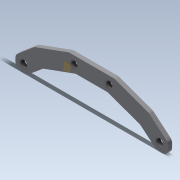
# Autodesk Inventor part: HeadTopConnector
Saved by Autodesk Inventor 2020 (Build 240168000, 168)
## iProperties
Created: 2021-07-09
Part Number: HeadTopConnector
Material: Generic
Document SubType Name: Sheet Metal
Designer: Val
Density: 1 g/cm^3
Sheet Metal Rule: Default
Appearance: Default
Author: Val
Autodesk Inventor part; units mm, degrees
ref_plane "YZ Plane" through (0, 0, 0) normal (1, 0, 0) x (0, 1, 0)
ref_plane "XZ Plane" through (0, 0, 0) normal (0, 1, 0) x (-1, 0, 0)
ref_plane "XY Plane" through (0, 0, 0) normal (0, 0, 1) x (1, 0, 0)
sketch "Base" plane through (0, 0, 0) normal (0, 0, 1) x (1, 0, 0)
  circle A0 centre (-46.4246, 117.9827) radius 2.5
  line L0 (-52.4246, 120.7805) -> (-52.4246, 111.9827)
  line L1 (-52.4246, 111.9827) -> (-44.2408, 111.9827)
  line L2 (-52.4246, 120.7805) -> (-44.8558, 127.1315)
  line L3 (-44.8558, 127.1315) -> (-16.5235, 137.4436)
  line L4 (-44.2408, 111.9827) -> (-38.7633, 116.5789)
  line L5 (-38.7633, 116.5789) -> (-11.6601, 126.4436)
  line L6 (-11.6601, 126.4436) -> (0.0157, 126.4436)
  line L7 (-16.5235, 137.4436) -> (0, 137.4436)
  line L8 (0.0001, 252.4162) -> (0.0001, -227.6975)
  line L9 (52.4249, 120.7805) -> (52.4249, 111.9827)
  line L10 (52.4249, 111.9827) -> (44.2411, 111.9827)
  line L11 (52.4249, 120.7805) -> (44.8561, 127.1315)
  line L12 (44.2411, 111.9827) -> (38.7635, 116.5789)
  line L13 (38.7635, 116.5789) -> (11.6604, 126.4436)
  line L14 (11.6604, 126.4436) -> (0.0157, 126.4436)
  line L15 (16.5238, 137.4436) -> (0, 137.4436)
  line L16 (16.5238, 137.4436) -> (44.8561, 127.1315)
  ellipse E0 centre (-12.7181, 132.4436) end of major axis (-10.7181, 132.4436) minor radius 1.9897
  ellipse E1 centre (12.7183, 132.4436) end of major axis (14.7183, 132.4436) minor radius 1.9897
  circle A1 centre (-46.4246, 117.9827) radius 3.175
  circle A2 centre (46.4246, 117.9827) radius 3.175
  point P0 (0, 0)
  dimension "d1" = 5
  dimension "d2" = 6
  dimension "d3" = 6
  dimension "d5" = 12
  dimension "d6" = 160
  dimension "d7" = 160
  dimension "d8" = 6
  dimension "d9" = 6
  dimension "d10" = 6
  dimension "d11" = 6
  dimension "d20" = 5
  measures "d1" distance from line of L7 E0.centre
  measures "d2" distance from line of L3 E0.centre
  measures "d3" distance from line of L6 E0.centre
  measures "d5" distance between parallel lines of L5 L3
  measures "d6" angle of L5 L4
  measures "d7" angle of L6 L5
  measures "d8" distance from line of L0 A0.centre
  measures "d9" distance from line of L2 A0.centre
  measures "d10" distance from line of L4 A0.centre
  measures "d11" distance from line of L1 A0.centre
  measures "d20" diameter of A0
extrude "Plate1" add sketch "Base" along normal blind 3.048 contours L2 L3 L7 L8 L6 L5 L4 L1 L0 | L15 L16 L11 L9 L10 L12 L13 L14 L6 L8
fillet "FilletsFeature" radius 4 14 edges at (-44.8558, 127.1315, 1.524) (-16.5235, 137.4436, 1.524) (-52.4246, 120.7805, 1.524) (-52.4246, 111.9827, 1.524) (16.5238, 137.4436, 1.524) (44.8561, 127.1315, 1.524) (52.4249, 120.7805, 1.524) (52.4249, 111.9827, 1.524) (44.2411, 111.9827, 1.524) (38.7635, 116.5789, 1.524) (11.6604, 126.4436, 1.524) (-11.6601, 126.4436, 1.524) (-38.7633, 116.5789, 1.524) (-44.2408, 111.9827, 1.524)
ref_plane "BentCutPlane" through (-12.7181, 132.4436, 8.3161) normal (0, 0.1014104, 0.9948447) x (0, -0.9948447, 0.1014104)
sketch "BentCutProfile" plane through (-12.7181, 132.4436, 8.3161) normal (0, 0.1014104, 0.9948447) x (0, -0.9948447, 0.1014104)
  circle A0 centre (0, 0) radius 2 projected
  circle A1 centre (0, 25.4364) radius 2 projected
  point P0 (130.9175, 12.7181)
hole "BentCutProfileHoleFeature" at (-12.7181, 132.4436, 8.3161) at (12.7183, 132.4436, 8.3161) direction (0, -0.1014104, -0.9948447) diameter 4.5 end through all
equation "\"d18\" = Thickness"
equation "\"d0\" = Thickness"
equation "\"BendRadius\" = Thickness"
equation "\"BendReliefWidth\" = Thickness"
equation "\"BendReliefDepth\" = 0.5 * Thickness"
equation "\"CornerReliefSize\" = 4 * Thickness"
equation "\"MinimumRemnant\" = 2 * Thickness"
equation "\"TransitionRadius\" = BendRadius"
equation "\"JacobiRadiusSize\" = BendRadius"
equation "\"GapSize\" = Thickness"
equation "\"Thickness\" = 3.048"
body "Solid1"
